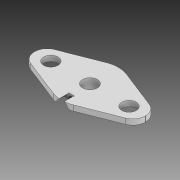
# Autodesk Inventor part: HD_rotor
Saved by Autodesk Inventor 2020 (Build 240168000, 168)
## iProperties
Created: 2021-03-19
Part Number: HD_rotor
Material: Generic
Document SubType Name: Modeling
Designer: DDeGo
Density: 1 g/cm^3
Appearance: Default
Author: DDeGo
Autodesk Inventor part; units mm, degrees
ref_plane "YZ Plane" through (0, 0, 0) normal (1, 0, 0) x (0, 1, 0)
ref_plane "XZ Plane" through (0, 0, 0) normal (0, 1, 0) x (-1, 0, 0)
ref_plane "XY Plane" through (0, 0, 0) normal (0, 0, 1) x (1, 0, 0)
sketch "608 bearing" plane through (0, 0, 0) normal (0, 0, 1) x (1, 0, 0)
  line L0 (-83.9037, 39.6189) -> (-76.9037, 39.6189) construction
  line L1 (-61.9037, 39.6189) -> (-61.9037, 32.6189) construction
  line L2 (-61.9037, 32.6189) -> (-68.9037, 32.6189) construction
  line L3 (-83.9037, 32.6189) -> (-83.9037, 39.6189) construction
  line L4 (-76.9037, 39.6189) -> (-76.9037, 32.6189) construction
  line L5 (-68.9037, 39.6189) -> (-68.9037, 32.6189) construction
  line L6 (-68.9037, 39.6189) -> (-61.9037, 39.6189) construction
  line L7 (-76.9037, 39.6189) -> (-68.9037, 39.6189) construction
  line L8 (-76.9037, 32.6189) -> (-83.9037, 32.6189) construction
  line L9 (-68.9037, 32.6189) -> (-76.9037, 32.6189) construction
  point P0 (-72.9037, 36.1189)
  point P1 (-72.9037, 39.6189)
  point P2 (-72.9037, 32.6189)
  dimension "d24" = 7
  dimension "d25" = 22
  dimension "d26" = 8
  measures "d24" distance of L1.start L1.end
  measures "d25" distance between parallel lines of L1 L3
  measures "d26" distance between parallel lines of L5 L4
derived "HD_mastersketch.ipt"
sketch "Belt" plane through (0, 0, 0) normal (0, 0, 1) x (1, 0, 0)
  line L0 (-33.9, 7.5) -> (-32.7, 7.5)
  line L1 (-32.7, 7.5) -> (-32.7, -7.5)
  line L2 (-32.7, -7.5) -> (-33.9, -7.5)
  line L3 (-33.9, -7.5) -> (-33.9, 7.5)
  point P0 (0, 0)
  point P1 (-33.9, 0)
sketch "Rotor" plane through (0, 0, 0) normal (0, 0, 1) x (1, 0, 0)
  line L0 (0, 0) -> (0, -29.5)
  line L1 (0, -29.5) -> (-4.075, -29.5)
  line L2 (-4.075, -29.5) -> (-4.075, -4.5)
  line L3 (-11.3123, -1.5) -> (-30.7, -1.5)
  line L4 (-30.7, -1.5) -> (-30.7, 1.5)
  line L5 (-30.7, 1.5) -> (-9.15, 1.5)
  line L6 (-4.075, 1.5) -> (-4.075, -4.5)
  line L7 (-4.075, 1.5) -> (-4.075, 13.5)
  line L8 (-4.075, 13.5) -> (0, 13.5)
  line L9 (0, 13.5) -> (0, 0)
  line L10 (-32.7, 7.5) -> (-32.7, -7.5) construction
  line L11 (-32.7, 0) -> (-30.7, 0) construction
  line L12 (-21.65, -2) -> (-21.65, -1.5) construction
  line L13 (-21.65, -1.5) -> (-21.65, 1.5) construction
  line L14 (-21.65, 2) -> (-21.65, 1.5) construction
  line L15 (-25.7, 1.5) -> (-25.7, -1.5) construction
  line L16 (-17.6, -1.5) -> (-17.6, 1.5) construction
  line L17 (-9.15, 1.5) -> (-9.15, -1.5) construction
  line L18 (-8.4662, -3.5513) -> (-8.15, -4.5)
  line L19 (-8.15, -4.5) -> (-4.075, -4.5)
  line L20 (-9.15, 1.5) -> (-8.15, 1.5)
  line L21 (-8.15, 1.5) -> (-8.15, -4.5) construction
  line L22 (-8.15, 1.5) -> (-4.075, 1.5)
  line L23 (-25.7, 0) -> (-21.65, 0) construction
  line L24 (-21.65, 0) -> (-17.6, 0) construction
  arc A0 (-8.4662, -3.5513) -> (-11.3123, -1.5) centre (-11.3123, -4.5) ccw
  line L25 (-32.65, 9) -> (-25.65, 9) construction
  line L26 (-10.65, 9) -> (-10.65, 2) construction
  line L27 (-10.65, 2) -> (-17.65, 2) construction
  line L28 (-32.65, 2) -> (-32.65, 9) construction
  line L29 (-25.65, 9) -> (-25.65, 2) construction
  line L30 (-17.65, 9) -> (-17.65, 2) construction
  line L31 (-17.65, 9) -> (-10.65, 9) construction
  line L32 (-25.65, 9) -> (-17.65, 9) construction
  line L33 (-25.65, 2) -> (-32.65, 2) construction
  line L34 (-17.65, 2) -> (-25.65, 2) construction
  line L35 (-32.65, -2) -> (-25.65, -2) construction
  line L36 (-10.65, -2) -> (-10.65, -9) construction
  line L37 (-10.65, -9) -> (-17.65, -9) construction
  line L38 (-32.65, -9) -> (-32.65, -2) construction
  line L39 (-25.65, -2) -> (-25.65, -9) construction
  line L40 (-17.65, -2) -> (-17.65, -9) construction
  line L41 (-17.65, -2) -> (-10.65, -2) construction
  line L42 (-25.65, -2) -> (-17.65, -2) construction
  line L43 (-25.65, -9) -> (-32.65, -9) construction
  line L44 (-17.65, -9) -> (-25.65, -9) construction
sketch "Base" plane through (0, 0, 0) normal (0, 0, 1) x (1, 0, 0)
  line L0 (0, -14.2) -> (-8.1, -14.2) construction
  line L1 (-40, -13.2) -> (-40, -1.25)
  line L2 (-39, -0.25) -> (-34, -0.25)
  line L3 (-27.65, -11.5) -> (-15.65, -11.5)
  line L4 (-10.15, -10) -> (-9.1, -6.2)
  line L5 (-9.1, -6.2) -> (-7.1, -6.2)
  line L6 (-7.1, -6.2) -> (-7.1, -7.7)
  line L7 (-7.1, -7.7) -> (-8.1, -8.7)
  line L8 (-8.1, -8.7) -> (-8.1, -14.2)
  line L9 (-8.1, -14.2) -> (-39, -14.2)
  line L10 (0, -14.2) -> (0, 38.4357) construction
  line L11 (-34, -0.25) -> (-34, -8)
  line L12 (-34, -8) -> (-32.5, -10)
  line L13 (-27.65, -10) -> (-27.65, -11.5)
  line L14 (-39, -0.25) -> (-40, -1.25)
  line L15 (-40, -13.2) -> (-39, -14.2)
  line L16 (-15.65, -11.5) -> (-15.65, -10)
  line L17 (-15.65, -10) -> (-10.15, -10)
  line L18 (-32.5, -10) -> (-27.65, -10)
  line L19 (0, 0) -> (-64.9444, 0) construction
  line L20 (-15.65, 11.5) -> (-15.65, 10)
  line L21 (-15.65, 10) -> (-10.15, 10)
  line L22 (-10.15, 10) -> (-9.1, 5)
  line L23 (-9.1, 5) -> (-7.1, 5)
  line L24 (-8.1, 7.5) -> (-8.1, 13)
  line L25 (-7.1, 5) -> (-7.1, 6.5)
  line L26 (-7.1, 6.5) -> (-8.1, 7.5)
  line L27 (0.103, 13) -> (-8.1, 13) construction
  line L28 (-27.65, 11.5) -> (-15.65, 11.5)
  line L29 (-8.1, 13) -> (-36.45, 13)
  line L30 (-37.45, 12) -> (-37.45, 1.25)
  line L31 (-38.45, 0.25) -> (-34, 0.25)
  line L32 (-27.65, 10) -> (-27.65, 11.5)
  line L33 (-32.5, 10) -> (-27.65, 10)
  line L34 (-34, 8) -> (-32.5, 10)
  line L35 (-34, 0.25) -> (-34, 8)
  line L36 (-37.45, 12) -> (-36.45, 13)
  line L37 (-38.45, 0.75) -> (-37.45, 1.25)
  line L38 (-33.9, -7.5) -> (-33.9, 7.5) construction
  line L39 (-32.7, -7.5) -> (-33.9, -7.5) construction
  line L40 (-21.65, -9) -> (-21.65, -11.5) construction
  line L41 (-30, 13) -> (-30, 12) construction
  line L42 (-30, 12) -> (-30, 10) construction
  line L43 (-30, -14.2) -> (-30, -12) construction
  line L44 (-25.65, -9) -> (-32.65, -9) construction
  line L45 (-8.15, -4.5) -> (-4.075, -4.5)
  line L46 (-8.15, 1.5) -> (-4.075, 1.5)
  line L47 (-8.1, 7.5) -> (-8.1, -8.7) construction
  line L48 (-38.45, 0.75) -> (-38.45, 0.25)
  line L49 (-30, -12) -> (-30, -10) construction
  point P0 (-40, -14.2)
  point P1 (-40, -0.25)
  point P2 (-37.45, 13)
  point P3 (-37.45, 0.25)
  point P4 (-21.65, 11.5)
revolve "Revolution1" add sketch "Rotor" angle 360 about axis through (0, 13.5, 0) along (0, -1, 0) contours L19 L18 A0 L3 L4 L5 L20 L22 L6
sketch "Sketch8" plane through (0, 1.5, 0) normal (0, 1, 0) x (1, 0, 0)
  circle A0 centre (0, 0) radius 30.7 projected
  line L0 (-30.2901, -5) -> (-5.7244, -14.6192)
  line L1 (-30.2901, -5) -> (-30.2901, 5) construction
  line L2 (-30.2901, 5) -> (-5.7244, 14.6192)
  circle A1 centre (0, 0) radius 4 construction
  line L3 (5.7244, -14.6192) -> (30.2901, -5)
  line L4 (30.2901, -5) -> (30.2901, 5) construction
  line L5 (30.2901, 5) -> (5.7244, 14.6192)
  arc A2 (-5.7244, -14.6192) -> (5.7244, -14.6192) centre (0, 0) ccw
  arc A3 (5.7244, 14.6192) -> (-5.7244, 14.6192) centre (0, 0) ccw
  point P0 (0, 0)
  dimension "d4" = 10
  dimension "d5" = 15
  constraints: 12 end point, 8 point on circle, 3 equal length, 2 centre point, 2 tangent, 2 vertical, 1 coincident, 1 concentric
  measures "d4" distance of L0.start L1.end
  measures "d5" radial gap between concentric circles of A0 A2
extrude "Extrusion1" cut sketch "Sketch8" against normal through all contours L5 A3 L2 A0 | A0 L0 A2 L3
sketch "Sketch9" plane through (0, 1.5, 0) normal (0, 1, 0) x (1, 0, 0)
  circle A0 centre (-21.65, 0) radius 4
  circle A1 centre (21.65, 0) radius 4
  circle A2 centre (0, 0) radius 16.1459 projected
  circle A3 centre (0, 0) radius 4.075 projected
  line L0 (0, 0) -> (0, 28.0271) construction
  point P0 (-25.65, 0)
  constraints: 2 end point, 1 centre point, 1 coincident, 1 horizontal alignment, 1 vertical, 3 other
extrude "Extrusion2" cut sketch "Sketch9" against normal through all contours A0 | A1
fillet "Fillet1" radius 7 4 edges at (30.2901, 0, 5) (30.2901, 0, -5) (-30.2901, 0, -5) (-30.2901, 0, 5)
sketch "Sketch10" plane through (0, -4.5, 0) normal (0, 1, 0) x (1, 0, 0)
  line L0 (-2.9, -6.2) -> (2.9, -6.2)
  line L1 (2.9, -6.2) -> (2.9, -3.7)
  line L2 (2.9, -3.7) -> (-2.9, -3.7)
  line L3 (-2.9, -3.7) -> (-2.9, -6.2)
  line L4 (-2.9, -6.2) -> (2.9, -3.7) construction
  line L5 (2.9, -6.2) -> (-2.9, -3.7) construction
  line L6 (0, 0) -> (0, -4.95) construction
  dimension "d11" = 3.7
  dimension "d12" = 2.5
  dimension "d13" = 5.8
  constraints: 14 end point, 2 midpoint, 2 parallel, 1 horizontal, 1 perpendicular, 1 vertical
  measures "d11" distance from line of L6.start L2
  measures "d12" distance of L0.end L1.end
  measures "d13" distance of L0.start L0.end
extrude "Extrusion3" cut sketch "Sketch10" along normal blind 5.8
sketch "Sketch14" plane through (0, 0, 0) normal (1, 0, 0) x (0, 1, 0)
  line L0 (-1.152, 6.2) -> (-1.152, 28.5259)
  line L1 (-1.152, 6.2) -> (0.498, 6.2)
  line L2 (0.498, 6.2) -> (0.498, 10.2)
  line L3 (0.498, 10.2) -> (1.848, 10.2)
  line L4 (1.848, 10.2) -> (1.848, 20.2)
  line L5 (1.848, 20.2) -> (0.348, 20.2)
  line L6 (0.348, 20.2) -> (0.348, 28.5259)
  line L7 (0.348, 28.5259) -> (-1.152, 28.5259)
  line L8 (-4.5, 6.2) -> (1.3, 6.2) projected
  point P0 (0, 0)
  point P1 (1.5, 0)
  point P2 (-3.604, 6.2)
  dimension "d29" = 1.65
  dimension "d30" = 3
  dimension "d32" = 10
  dimension "d33" = 1.5
  dimension "d36" = 4
  constraints: 16 end point, 5 perpendicular, 2 vertical, 1 horizontal, 1 point on line
  measures "d29" distance between parallel lines of L0 L2
  measures "d30" distance between parallel lines of L0 L4
  measures "d32" distance of L3.end L4.end
  measures "d33" distance between parallel lines of L0 L6
  measures "d36" distance between parallel lines of L8 L3
revolve "Revolution2" cut sketch "Sketch14" angle 360 about axis through (0, -1.152, 6.2) along (0, 0, 1)
fillet "Fillet3" radius 2 2 edges at (2.9773, -1.5199, 10.555) (-2.9773, -1.5199, 10.555)
body "Solid1"
